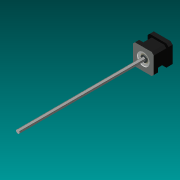
# Autodesk Inventor part: 步进电机
Saved by Autodesk Inventor 2021 (Build 250183000, 183)
## iProperties
Created: 2025-04-17
Part Number: 步进电机
Material: 常规
Document SubType Name: Modeling
Designer: 86155
Density: 1 g/cm^3
Appearance: 默认
Author: 86155
Autodesk Inventor part; units mm, degrees
ref_plane "YZ Plane" through (0, 0, 0) normal (1, 0, 0) x (0, 1, 0)
ref_plane "XZ Plane" through (0, 0, 0) normal (0, 1, 0) x (-1, 0, 0)
ref_plane "XY Plane" through (0, 0, 0) normal (0, 0, 1) x (1, 0, 0)
sketch "草图1" plane through (0, 0, 0) normal (0, 0, 1) x (1, 0, 0)
  circle A0 centre (0, 0) radius 4.25
  dimension "d0" = 8.5
  constraints: 1 centre point, 1 coincident
  measures "d0" diameter of A0
extrude "拉伸1" add sketch "草图1" along normal blind 450
sketch "草图2" plane through (0, 0, 0) normal (0, 0, -1) x (-1, 0, 0)
  line L0 (-25, 25) -> (25, 25)
  line L1 (25, 25) -> (25, -25)
  line L2 (25, -25) -> (-25, -25)
  line L3 (-25, -25) -> (-25, 25)
  circle A0 centre (0, 0) radius 4.25 projected
  line L4 (-25, 25) -> (25, -25) construction
  line L5 (25, 25) -> (-25, -25) construction
  dimension "d3" = 50
  dimension "d4" = 50
  constraints: 12 end point, 2 midpoint, 2 parallel, 1 horizontal, 1 perpendicular
  measures "d3" distance of L1.end L2.end
  measures "d4" distance of L0.end L1.end
extrude "拉伸2" add sketch "草图2" along normal blind 10 contours L0 L1 L2 L3 | A0
sketch "草图3" plane through (0, 0, 0) normal (0, 0, 1) x (1, 0, 0)
  circle A0 centre (0, 0) radius 15
  dimension "d7" = 30
  constraints: 1 centre point, 1 coincident
  measures "d7" diameter of A0
extrude "拉伸3" cut sketch "草图3" against normal blind 2
sketch "草图4" plane through (0, 0, -2) normal (0, 0, 1) x (1, 0, 0)
  circle A0 centre (0, 0) radius 10
  dimension "d10" = 20
  constraints: 1 centre point, 1 coincident
  measures "d10" diameter of A0
extrude "拉伸4" cut sketch "草图4" against normal blind 1
sketch "草图5" plane through (0, 0, -3) normal (0, 0, 1) x (1, 0, 0)
  circle A0 centre (0, 0) radius 7.5
  dimension "d13" = 15
  constraints: 1 centre point, 1 coincident
  measures "d13" diameter of A0
extrude "拉伸5" add sketch "草图5" along normal blind 2
sketch "草图6" plane through (0, 0, -1) normal (0, 0, 1) x (1, 0, 0)
  circle A0 centre (0, 0) radius 4.25 projected
extrude "拉伸6" add sketch "草图6" along normal blind 2
sketch "草图7" plane through (0, 0, -10) normal (0, 0, -1) x (-1, 0, 0)
  line L0 (-20, 20) -> (20, 20)
  line L1 (20, 20) -> (20, -20)
  line L2 (20, -20) -> (-20, -20)
  line L3 (-20, -20) -> (-20, 20)
  line L4 (-20, 20) -> (20, -20) construction
  line L5 (20, 20) -> (-20, -20) construction
  point P0 (0, 0)
  dimension "d18" = 40
  dimension "d19" = 40
  constraints: 12 end point, 2 midpoint, 2 parallel, 1 horizontal, 1 perpendicular
  measures "d18" distance of L1.end L2.end
  measures "d19" distance of L0.end L1.end
extrude "拉伸7" add sketch "草图7" along normal blind 25
sketch "草图8" plane through (0, 0, -35) normal (0, 0, -1) x (-1, 0, 0)
  line L0 (25, -25) -> (25, 25) projected
  line L1 (-25, 25) -> (25, 25)
  line L2 (25, 25) -> (25, -25)
  line L3 (25, -25) -> (-25, -25)
  line L4 (-25, -25) -> (-25, 25)
  circle A0 centre (0, 0) radius 7.5 projected
  line L5 (-25, 25) -> (25, -25) construction
  line L6 (25, 25) -> (-25, -25) construction
  dimension "d22" = 50
  dimension "d23" = 50
  constraints: 12 end point, 2 midpoint, 2 parallel, 1 horizontal, 1 perpendicular
  measures "d22" distance of L0.start L3.end
  measures "d23" distance of L1.end L0.start
extrude "拉伸8" add sketch "草图8" along normal blind 10 contours L3 L4 L1 L0 | A0
chamfer "倒角1" distance 5 angle 45 12 edges at (20, -20, -22.5) (25, -25, -5) (25, -25, -40) (-25, -25, -40) (-20, -20, -22.5) (-25, -25, -5) (25, 25, -5) (20, 20, -22.5) (25, 25, -40) (-20, 20, -22.5) (-25, 25, -5) (-25, 25, -40)
thread "螺纹1" size "M9x1.25" class "6g" standard "ANSI Metric M Profile" full length
